Autodesk Fusion 360 part; units mm, degrees
note: some values were not read from the file. Set by a fixed rule: which sketch regions a step uses.
(part 2 of 2)
sketch "Topbase.dxf" plane through (0, 0, 0) normal (0, 0, -1) x (1, 0, 0)
  line L0 (149.286, 3) -> (146.286, 3)
  line L1 (146.286, 3) -> (146.286, 83)
  line L2 (146.286, 83) -> (149.286, 83)
  line L3 (149.286, 83) -> (149.286, 3)
  line L4 (37.3742, 85.4546) -> (37.3742, 82.4546)
  line L5 (37.3742, 82.4546) -> (20.1905, 82.4546)
  line L6 (20.1905, 82.4546) -> (20.1905, 85.4546)
  line L7 (20.1905, 85.4546) -> (37.3742, 85.4546)
  line L8 (71.7416, 85.4546) -> (71.7416, 82.4546)
  line L9 (71.7416, 82.4546) -> (54.5579, 82.4546)
  line L10 (54.5579, 82.4546) -> (54.5579, 85.4546)
  line L11 (54.5579, 85.4546) -> (71.7416, 85.4546)
  line L12 (106.109, 85.4546) -> (106.109, 82.4546)
  line L13 (106.109, 82.4546) -> (88.9253, 82.4546)
  line L14 (88.9253, 82.4546) -> (88.9253, 85.4546)
  line L15 (88.9253, 85.4546) -> (106.109, 85.4546)
  line L16 (123.286, 35) -> (126.286, 35)
  line L17 (126.286, 35) -> (126.286, 19)
  line L18 (126.286, 19) -> (123.286, 19)
  line L19 (123.286, 19) -> (123.286, 35)
  line L20 (123.286, 67) -> (126.286, 67)
  line L21 (126.286, 67) -> (126.286, 51)
  line L22 (126.286, 51) -> (123.286, 51)
  line L23 (123.286, 51) -> (123.286, 67)
  line L24 (0, 35) -> (3, 35)
  line L25 (3, 35) -> (3, 19)
  line L26 (3, 19) -> (0, 19)
  line L27 (0, 19) -> (0, 35)
  line L28 (0, 67) -> (3, 67)
  line L29 (3, 67) -> (3, 51)
  line L30 (3, 51) -> (0, 51)
  line L31 (0, 51) -> (0, 67)
  line L32 (88.9186, 0) -> (88.9186, 3)
  line L33 (88.9186, 3) -> (106.1023, 3)
  line L34 (106.1023, 3) -> (106.1023, 0)
  line L35 (106.1023, 0) -> (88.9186, 0)
  line L36 (54.5511, 0) -> (54.5511, 3)
  line L37 (54.5511, 3) -> (71.7349, 3)
  line L38 (71.7349, 3) -> (71.7349, 0)
  line L39 (71.7349, 0) -> (54.5511, 0)
  line L40 (20.1837, 0) -> (20.1837, 3)
  line L41 (20.1837, 3) -> (37.3674, 3)
  line L42 (37.3674, 3) -> (37.3674, 0)
  line L43 (37.3674, 0) -> (20.1837, 0)
  line L44 (-25, 96) -> (-25, -10)
  line L45 (-25, -10) -> (175, -10)
  line L46 (175, -10) -> (175, 96)
  line L47 (175, 96) -> (-25, 96)
component "Back" placed x (1, 0, 0) y (0, 1, 0) z (0, 0, 1) at (0, 0, 0)
component "left" placed x (1, 0, 0) y (0, 1, 0) z (0, 0, 1) at (0, 0, 0)
component "Front" placed x (1, 0, 0) y (0, 1, 0) z (0, 0, 1) at (0, 0, 0)
component "lid" placed x (1, 0, 0) y (0, 1, 0) z (0, 0, 1) at (0, 0, 0)
component "Top Base" placed x (1, 0, 0) y (0, 1, 0) z (0, 0, 1) at (0, 0, 0)
equation "length = 120.286 mm"
equation "width = 80 mm"
equation "height = 70 mm"
equation "thickness = 3 mm"
equation "lfinger = 3" comment "number of fingers for length"
equation "hfinger = 3" comment "number of fingers for height"
equation "wfinger = 2" comment "number of fingers for width"
equation "d10 = thickness"
equation "d11 = height / ( 2 * hfinger + 1 )"
equation "d13 = d11"
equation "d14 = d13"
equation "d15 = d14"
equation "d18 = -thickness"
equation "d24 = height / ( 2 * hfinger + 1 )"
equation "d25 = d24"
equation "d26 = d25"
equation "d27 = d26"
equation "d28 = d27"
equation "d45 = thickness"
equation "d58 = thickness"
equation "d59 = ( length / ( lfinger * 2 ) + 1 mm )"
equation "d60 = d59"
equation "d61 = d60"
equation "d63 = d61"
equation "d67 = thickness"
equation "d68 = width / ( wfinger * 2 + 1 )"
equation "d69 = d68"
equation "d70 = d69"
equation "d98 = thickness"
equation "d99 = thickness"
equation "d101 = thickness"
equation "d103 = thickness"
equation "d109 = thickness"
equation "d111 = thickness"
equation "d114 = thickness"
equation "d137 = thickness"
equation "d140 = thickness"
equation "d141 = thickness"
equation "d142 = thickness"
equation "d150 = length / ( 2 * lfinger + 1 )"
equation "d151 = d150"
equation "d153 = d151"
equation "d154 = d153"
equation "d155 = d154"
equation "d156 = d155"
equation "d157 = d156"
equation "d159 = thickness"
equation "d161 = thickness"
equation "d162 = height / ( 2 * hfinger + 1 )"
equation "d166 = d162"
equation "d167 = d166"
equation "d169 = thickness"
equation "d171 = height"
equation "d172 = length"
equation "d173 = length / ( 2 * lfinger + 1 )"
equation "d174 = d173"
equation "d175 = d174"
equation "d176 = d175"
equation "d177 = d176"
equation "d178 = d177"
equation "d180 = width / ( wfinger * 2 + 1 )"
equation "d181 = d180"
equation "d182 = d181"
equation "d183 = d182"
equation "d185 = width"
equation "d187 = height"
equation "d188 = height / ( hfinger * 2 + 1 )"
equation "d189 = d188"
equation "d191 = d190"
equation "d192 = d191"
equation "d193 = d192"
equation "d195 = height"
equation "d196 = d167"
equation "d197 = d196"
equation "d198 = d197"
equation "d200 = height / ( hfinger * 2 + 1 )"
equation "d201 = d200"
equation "d202 = d201"
equation "d203 = d202"
equation "d204 = d203"
equation "d205 = d204"
equation "d207 = length"
equation "d208 = width"
equation "d209 = length"
equation "d212 = 200 mm - 25 mm"
equation "d217 = thickness"
equation "d219 = thickness"
equation "d222 = -thickness"
equation "d224 = length / ( 2 * lfinger + 1 )"
equation "d225 = d224"
equation "d226 = d225"
equation "d227 = d226"
equation "d228 = d227"
equation "d229 = d228"
